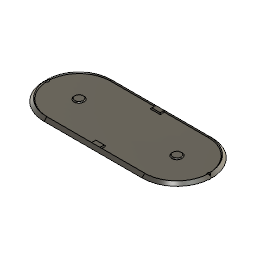
Controller cover (Autodesk Fusion 360 design; units mm, degrees)
part number: 2026-01-06-17-29-56-403
Autodesk Fusion 360 part; units mm, degrees
note: some values were not read from the file. Set by a fixed rule: which sketch regions a step uses.
sketch "Skizze1" plane through (0, 0, 0) normal (0, 0, 1) x (1, 0, 0)
  line L0 (0, 0) -> (70, 0)
  line L1 (70, 0) -> (70, -50)
  line L2 (70, -50) -> (0, -50)
  line L3 (0, -50) -> (0, 0)
  circle A0 centre (0, -25) radius 25
  circle A1 centre (70, -25) radius 25
  dimension "d1" = 70
  dimension "d2" = 50
  constraint horizontal L0
  constraint vertical L1
  constraint horizontal L2
  constraint vertical L3
  constraint coincident L0.start L3.end
  constraint midpoint L3 A0.centre
  constraint coincident L0.start A0
  constraint midpoint L1 A1.centre
  constraint coincident L0.end A1
  measures "d1" distance of L0.start L0.end
  measures "d2" distance of L0.start L2.end
extrude "Extrusion1" add sketch "Skizze1" along normal blind 2 draft -45
hole "Bohrung1" at (-23, -25, 2) direction (0, 0, -1) diameter 1.5 depth 2 tip angle 180
hole "Bohrung2" at (93, -25, 2) direction (0, 0, -1) diameter 1.5 depth 2 tip angle 180
fillet "Abrundung1" radius 1 curvature continuous tangency weight 0.1 2 edges at (92.3008, -25.2712, 0) (-23.6992, -25.2712, 0)
sketch "Skizze2" plane through (0, 0, 2) normal (0, 0, 1) x (-1, 0, 0)
  arc A0 (-92.9878, 24.2501) -> (-92.9878, 25.7499) centre (-93, 25) ccw
  arc A1 (-92.9878, 24.2501) -> (-70, 2) centre (-70, 25) ccw
  line L0 (-70, 2) -> (0, 2)
  arc A2 (0, 2) -> (22.9878, 24.2501) centre (0, 25) ccw
  arc A3 (22.9878, 25.7499) -> (22.9878, 24.2501) centre (23, 25) ccw
  arc A4 (22.9878, 25.7499) -> (0, 48) centre (0, 25) ccw
  line L1 (0, 48) -> (-70, 48)
  arc A5 (-70, 48) -> (-92.9878, 25.7499) centre (-70, 25) ccw
  line L2 (0, 2) -> (-70, 2)
  line L3 (-70, 2) -> (-70, 48)
  line L4 (-70, 48) -> (0, 48)
  line L5 (0, 48) -> (0, 2)
  circle A6 centre (0, 25) radius 3
  circle A7 centre (-70, 25) radius 3
  line L6 (-32, 2) -> (-38, 2)
  line L7 (-38, 2) -> (-38, 5)
  line L8 (-38, 5) -> (-32, 5)
  line L9 (-32, 5) -> (-32, 2)
  line L10 (-32, 48) -> (-38, 48)
  line L11 (-38, 48) -> (-38, 45)
  line L12 (-38, 45) -> (-32, 45)
  line L13 (-32, 45) -> (-32, 48)
  dimension "d13" = 6
  dimension "d14" = 6
  dimension "d15" = 3
  constraint horizontal L2
  constraint vertical L3
  constraint horizontal L4
  constraint vertical L5
  constraint coincident L1.end A5.start
  constraint coincident L0.end A2.start
  constraint concentric A2 A6
  constraint concentric A1 A7
  constraint horizontal L6
  constraint vertical L7
  constraint horizontal L8
  constraint vertical L9
  constraint coincident L0 L6.start
  constraint horizontal L10
  constraint vertical L11
  constraint horizontal L12
  constraint vertical L13
  constraint coincident L1 L10.start
  measures "d13" diameter of A6
  measures "d14" diameter of A7
  measures "d15" distance of L6.start L8.end
extrude "Extrusion2" cut sketch "Skizze2" against normal blind 0.6 draft -45 contours A0 A1 A5 L3 A7 | L0 L1 L2 L3 L4 L5 A6 A7 L7 L8 L9 L11 L12 L13 | A2 A3 A4 L5 A6
